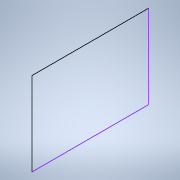
# Autodesk Inventor part: ロボットベースT5.5_2
Saved by Autodesk Inventor 2020.3 (Build 243373000, 373)
## iProperties
Created: 2020-07-24
Part Number: ロボットベースT5.5_2
Material: 木材 (オーク)
Document SubType Name: Modeling
Designer: totot
Density: 0.76 g/cm^3
Appearance: ホワイト オーク材 - ナチュラル 標準の光沢
Author: totot
Autodesk Inventor part; units mm, degrees
ref_plane "YZ Plane" through (0, 0, 0) normal (1, 0, 0) x (0, 1, 0)
ref_plane "XZ Plane" through (0, 0, 0) normal (0, 1, 0) x (-1, 0, 0)
ref_plane "XY Plane" through (0, 0, 0) normal (0, 0, 1) x (1, 0, 0)
sketch "スケッチ1" plane through (0, 0, 0) normal (1, 0, 0) x (0, 1, 0)
  line L0 (0, 0) -> (-110, 0)
  line L1 (-110, 0) -> (-110, -116)
  line L2 (-110, -116) -> (0, -116)
  line L3 (0, -116) -> (0, 0)
  dimension "d0" = 110
  dimension "d1" = 116
  constraints: 8 end point, 2 parallel, 1 horizontal, 1 perpendicular
  measures "d0" distance between parallel lines of L1 L3
  measures "d1" distance between parallel lines of L0 L2
extrude "押し出し1" add sketch "スケッチ1" along normal blind 5.5
fillet "フィレット1" radius 5 4 edges at (2.75, 0, 0) (2.75, 0, -116) (2.75, -110, 0) (2.75, -110, -116)
sketch "スケッチ2" plane through (5.5, 0, 0) normal (1, 0, 0) x (0, 0, -1)
  line L0 (7.5, -5) -> (108.5, -5)
  line L1 (108.5, -5) -> (108.5, -105)
  line L2 (108.5, -105) -> (7.5, -105)
  line L3 (7.5, -105) -> (7.5, -5)
  line L4 (111, 0) -> (5, 0) projected
  line L5 (0, -5) -> (0, -105) projected
  point P0 (0, 0)
  dimension "d5" = 101
  dimension "d6" = 100
  dimension "d7" = 5
  dimension "d8" = 7.5
  constraints: 8 end point, 4 coincident, 2 parallel, 1 horizontal, 1 perpendicular
  measures "d5" distance of L1.end L2.end
  measures "d6" distance of L0.end L1.end
  measures "d7" distance between parallel lines of L0 L4
  measures "d8" distance between parallel lines of L5 L3
hole "穴1" at (5.5, -5, -7.5) at (5.5, -5, -108.5) at (5.5, -105, -108.5) at (5.5, -105, -7.5) direction (-1, 0, 0) diameter 3 end through all
sketch "スケッチ3" plane through (5.5, 0, 0) normal (1, 0, 0) x (0, 0, -1)
  circle A0 centre (58, -88) radius 15
  line L0 (0, -5) -> (0, -105) projected
  line L1 (5, -110) -> (111, -110) projected
  point P0 (0, 0)
  dimension "d16" = 30
  dimension "d17" = 58
  dimension "d18" = 22
  constraints: 1 centre point
  measures "d16" diameter of A0
  measures "d17" distance from line of A0.centre L0
  measures "d18" distance from line of L1 A0.centre
extrude "押し出し2" cut sketch "スケッチ3" against normal through all
sketch "スケッチ4" plane through (5.5, 0, 0) normal (1, 0, 0) x (0, 0, -1)
  circle A0 centre (58, -22) radius 15
  line L0 (111, 0) -> (5, 0) projected
  circle A1 centre (58, -88) radius 15 projected
  line L1 (0, -5) -> (0, -105) projected
  point P0 (0, 0)
  dimension "d21" = 30
  dimension "d22" = 22
  dimension "d23" = 58
  dimension "d24" = 58
  constraints: 1 centre point
  measures "d21" diameter of A0
  measures "d22" distance from line of L0 A0.centre
  measures "d23" distance from line of A1.centre L1
  measures "d24" distance from line of L1 A0.centre
sketch "スケッチ5" plane through (5.5, 0, 0) normal (1, 0, 0) x (0, 0, -1)
  point P0 (0, 0)
extrude "押し出し3" cut sketch "スケッチ4" against normal through all contours A0
equation "\"d24\" = d23"
